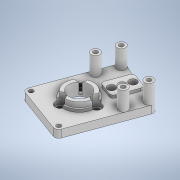
# Autodesk Inventor part: BASE_PLATE
Saved by Autodesk Inventor 2022 (Build 260153070, 153G)
## iProperties
Created: 2022-01-11
Part Number: BASE_PLATE
Material: Generic
Document SubType Name: Modeling
Designer: a laptop
Density: 1 g/cm^3
Appearance: Default
Author: a laptop
Autodesk Inventor part; units mm, degrees
ref_plane "YZ Plane" through (0, 0, 0) normal (1, 0, 0) x (0, 1, 0)
ref_plane "XZ Plane" through (0, 0, 0) normal (0, 1, 0) x (-1, 0, 0)
ref_plane "XY Plane" through (0, 0, 0) normal (0, 0, 1) x (1, 0, 0)
sketch "Sketch1" plane through (0, 0, 0) normal (0, 1, 0) x (-1, 0, 0)
  circle A0 centre (0, 0) radius 1.5
  circle A1 centre (-11.0608, 10.4718) radius 1.35 projected
  circle A2 centre (-15.2112, -0.7876) radius 1.35 projected
  circle A3 centre (11.0608, -10.4718) radius 1.35 projected
  circle A4 centre (15.2112, 0.7876) radius 1.35 projected
  line L0 (-13.5003, 11.3711) -> (-17.6507, 0.1117) projected
  line L1 (13.5003, -11.3711) -> (17.6507, -0.1117) projected
  arc A5 (-17.6507, 0.1117) -> (-15.7505, -3.331) centre (-15.2112, -0.7876) ccw projected
  arc A6 (-7.4411, -5.73) -> (-15.7505, -3.331) centre (-28.2044, -62.0577) ccw projected
  line L2 (-7.4411, -5.73) -> (1.9418, -9.1887) projected
  arc A7 (9.8203, -12.7568) -> (1.9418, -9.1887) centre (-18.8216, -65.5164) ccw projected
  arc A8 (9.8203, -12.7568) -> (13.5003, -11.3711) centre (11.0608, -10.4718) ccw projected
  circle A9 centre (-0.6847, 38.6203) radius 1.35
  circle A10 centre (25.5872, 28.936) radius 1.35
  line L3 (15.2112, 0.7876) -> (25.5872, 28.936) construction
  line L4 (25.5872, 28.936) -> (-0.6847, 38.6203) construction
  line L5 (-0.6847, 38.6203) -> (-11.0608, 10.4718) construction
  line L6 (-11.0608, 10.4718) -> (15.2112, 0.7876) construction
  circle A11 centre (-0.6847, 38.6203) radius 2.6
  circle A12 centre (25.5872, 28.936) radius 2.6
  line L7 (-13.5003, 11.3711) -> (-3.1243, 39.5196)
  line L8 (0.2145, 41.0599) -> (26.4865, 31.3756)
  line L9 (17.6507, -0.1117) -> (28.0267, 28.0368)
  circle A13 centre (6.9174, 18.7657) radius 6.25 projected
  dimension "d0" = 3
  dimension "d1" = 2.7
  dimension "d2" = 2.7
  dimension "d3" = 30
  dimension "d4" = 1.25
  constraints: 14 end point, 5 centre point, 5 coincident, 4 point on circle, 4 tangent, 2 perpendicular, 1 equal radius, 1 parallel
  measures "d0" diameter of A0
  measures "d1" diameter of A9
  measures "d2" diameter of A10
  measures "d3" distance between parallel lines of L6 L4
  measures "d4" radial gap between concentric circles of A9 A11
extrude "Extrusion1" add sketch "Sketch1" along normal blind 3
sketch "Sketch2" plane through (0, 0, 0) normal (0, -1, 0) x (1, 0, 0)
  circle A0 centre (-6.9174, 18.7657) radius 14.5
  circle A1 centre (-6.9174, 18.7657) radius 12 projected
  circle A2 centre (0, 0) radius 3.05
  circle A3 centre (0, 0) radius 1.5 projected
  line L0 (-1.7424, -2.5033) -> (-15.2011, 6.8649)
  line L1 (2.9503, -0.7734) -> (7.1087, 15.0886)
  circle A4 centre (-11.0608, -10.4718) radius 2.6
  circle A5 centre (-15.2112, 0.7876) radius 2.6
  circle A6 centre (-25.5872, 28.936) radius 2.6
  circle A7 centre (0.6847, 38.6203) radius 2.6
  circle A8 centre (11.0608, 10.4718) radius 2.6
  circle A9 centre (15.2112, -0.7876) radius 2.6
  circle A10 centre (-11.0608, -10.4718) radius 1.35 projected
  circle A11 centre (-15.2112, 0.7876) radius 1.35 projected
  circle A12 centre (-25.5872, 28.936) radius 1.35 projected
  circle A13 centre (0.6847, 38.6203) radius 1.35 projected
  circle A14 centre (11.0608, 10.4718) radius 1.35 projected
  circle A15 centre (15.2112, -0.7876) radius 1.35 projected
  circle A16 centre (1.7293, -4.6914) radius 1.15 projected
  circle A17 centre (-1.7293, 4.6914) radius 1.15 projected
  circle A18 centre (1.7293, -4.6914) radius 2.4
  arc A19 (7.1087, 15.0886) -> (4.1273, -4.7906) centre (97.7032, -8.6614) ccw
  arc A20 (-0.0305, -6.3233) -> (-15.2011, 6.8649) centre (-68.7061, -70.0029) ccw
  circle A21 centre (-6.9174, 18.7657) radius 12.35
  dimension "d7" = 2.5
  dimension "d8" = 6.1
  dimension "d10" = 1.25
  dimension "d13" = 1.25
  dimension "d14" = 0.35
  constraints: 12 centre point, 10 point on circle, 9 concentric, 8 tangent, 5 equal radius, 4 end point, 1 coincident
  measures "d7" radial gap between concentric circles of A0 A1
  measures "d8" diameter of A2
  measures "d10" radial gap between concentric circles of A4 A10
  measures "d13" radial gap between concentric circles of A16 A18
  measures "d14" radial gap between concentric circles of A1 A21
extrude "Extrusion2" add sketch "Sketch2" along normal blind 1.6 contours A0 A17 | A0 A17 L1 A2 L0 | L0 A2 A18 A20 | A19 A18 A2 L1 | A17 A0 | A0 A17 | A18 A2 | A4 | A5 | A6 | A7 | A8 | A9 | A16 picked at (3.6779, -4.407)
sketch "Sketch3" plane through (0, 3, 0) normal (0, 1, 0) x (1, 0, 0)
  circle A0 centre (-6.9174, -18.7657) radius 6.25 projected
  circle A1 centre (-6.9174, -18.7657) radius 9.5
  point P0 (0, 0)
  dimension "d15" = 19
  constraints: 1 centre point, 1 coincident
  measures "d15" diameter of A1
extrude "Extrusion3" add sketch "Sketch3" along normal blind 1.6
sketch "Sketch4" plane through (-6.9174, 4.6, 18.7657) normal (0, 1, 0) x (1, 0, 0)
  circle A0 centre (0, 0) radius 8.425
  circle A1 centre (0, 0) radius 6.25 projected
  point P0 (6.9174, 18.7657)
  dimension "d18" = 16.85
  constraints: 1 centre point, 1 concentric
  measures "d18" diameter of A0
extrude "Extrusion4" add sketch "Sketch4" along normal blind 3
sketch "Sketch5" plane through (-6.9174, 7.6, 18.7657) normal (0, 1, 0) x (1, 0, 0)
  circle A0 centre (-5.7568, 6.918) radius 1.6 projected
  circle A1 centre (-3.1128, -8.4445) radius 1.6 projected
  circle A2 centre (8.8696, 1.5265) radius 1.6 projected
  point P0 (6.9174, 18.7657)
extrude "Extrusion5" cut sketch "Sketch5" against normal up to surface (7.6 mm away)
sketch "Sketch6" plane through (-6.9174, 7.6, 18.7657) normal (0, 1, 0) x (1, 0, 0)
  circle A0 centre (-3.1128, -8.4445) radius 2.875
  circle A1 centre (-5.7568, 6.918) radius 2.875
  circle A2 centre (8.8696, 1.5265) radius 2.875
  arc A3 (-4.7015, -8.255) -> (-1.7812, -9.3315) centre (-3.1128, -8.4445) ccw projected
  arc A4 (-4.7983, 8.1992) -> (-7.1908, 6.2083) centre (-5.7568, 6.918) ccw projected
  arc A5 (9.4998, 0.0559) -> (8.9719, 3.1232) centre (8.8696, 1.5265) ccw projected
  point P0 (6.9174, 18.7657)
  dimension "d23" = 5.75
  constraints: 3 centre point, 3 concentric, 2 equal radius
  measures "d23" diameter of A1
extrude "Extrusion6" cut sketch "Sketch6" against normal blind 6.5
sketch "Sketch7" plane through (0, 3, 0) normal (0, 1, 0) x (1, 0, 0)
  circle A0 centre (0, 0) radius 1.875 projected
  circle A1 centre (1.7293, 4.6914) radius 1.15 projected
  circle A2 centre (-1.7293, -4.6914) radius 1.15 projected
  circle A3 centre (0, 0) radius 2.275
  line L0 (7.2185, 3.6805) -> (3.1891, -7.2505)
  line L1 (0.6208, -8.4353) -> (-5.9472, -6.0142)
  line L2 (-7.132, -3.4459) -> (-3.1026, 7.4851)
  line L3 (-0.5343, 8.6699) -> (6.0336, 6.2488)
  line L4 (7.4411, 5.73) -> (-1.9418, 9.1887) projected
  arc A4 (0.6208, -8.4353) -> (3.1891, -7.2505) centre (1.3125, -6.5588) ccw
  arc A5 (7.2185, 3.6805) -> (6.0336, 6.2488) centre (5.3419, 4.3722) ccw
  arc A6 (-0.5343, 8.6699) -> (-3.1026, 7.4851) centre (-1.2261, 6.7933) ccw
  arc A7 (-7.132, -3.4459) -> (-5.9472, -6.0142) centre (-5.2554, -4.1377) ccw
  dimension "d26" = 0.4
  dimension "d27" = 5.5
  dimension "d28" = 5.5
  dimension "d29" = 2.7
  dimension "d30" = 2
  constraints: 8 end point, 8 point on circle, 8 tangent, 5 centre point, 3 equal radius, 3 perpendicular, 1 collinear, 1 concentric, 1 point on line
  measures "d26" radial gap between concentric circles of A0 A3
  measures "d27" distance from line of L0 A3.centre
  measures "d28" distance from line of L2 point (0, 0)
  measures "d29" distance from line of A2.centre L1
  measures "d30" radius of A4
extrude "Extrusion7" add sketch "Sketch7" along normal blind 1.6 contours L0 A4 L1 A7 L2 A6 L3 A5
sketch "Sketch8" plane through (0, 4.6, 0) normal (0, 1, 0) x (1, 0, 0)
  circle A0 centre (1.7293, 4.6914) radius 2.3
  circle A1 centre (1.7293, 4.6914) radius 1.15 projected
  circle A2 centre (-1.7293, -4.6914) radius 2.3
  circle A3 centre (-1.7293, -4.6914) radius 1.15 projected
  point P0 (0, 0)
  dimension "d33" = 4.6
  dimension "d34" = 4.6
  constraints: 2 centre point, 2 concentric
  measures "d33" diameter of A0
  measures "d34" diameter of A2
extrude "Extrusion8" cut sketch "Sketch8" against normal blind 3.6 contours A0 | A1 | A2 | A3
sketch "Sketch9" plane through (-1.7293, 1, 4.6914) normal (0, 1, 0) x (1, 0, 0)
  circle A0 centre (0, 0) radius 1.15
  circle A1 centre (3.4587, 9.3828) radius 1.15
  circle A2 centre (3.4587, 9.3828) radius 2.3 projected
  circle A3 centre (0, 0) radius 2.3 projected
  point P0 (1.7293, 4.6914)
  dimension "d37" = 2.3
  constraints: 2 centre point, 2 concentric, 1 equal radius
  measures "d37" diameter of A1
extrude "Extrusion9" cut sketch "Sketch9" against normal blind 10 contours A0 | A1
sketch "Sketch10" plane through (0, 3, 0) normal (0, 1, 0) x (1, 0, 0)
  circle A0 centre (-11.0608, 10.4718) radius 2.6 projected
  circle A1 centre (-11.0608, 10.4718) radius 1.35 projected
  circle A2 centre (-15.2112, -0.7876) radius 2.6 projected
  circle A3 centre (-15.2112, -0.7876) radius 1.35 projected
  circle A4 centre (15.2112, 0.7876) radius 2.6 projected
  circle A5 centre (15.2112, 0.7876) radius 1.35 projected
  circle A6 centre (11.0608, -10.4718) radius 2.6 projected
  circle A7 centre (11.0608, -10.4718) radius 1.35 projected
  point P0 (0, 0)
extrude "Extrusion10" add sketch "Sketch10" along normal blind 11.32
sketch "Sketch11" plane through (-15.2112, 0, 0.7876) normal (0, -1, 0) x (1, 0, 0)
  arc A0 (15.1806, -7.1108) -> (0.0101, 6.0773) centre (-53.495, -70.7904) ccw projected
  arc A1 (22.3198, 14.3011) -> (0.0101, 6.0773) centre (8.2938, 17.9781) ccw projected
  arc A2 (22.3198, 14.3011) -> (19.3385, -5.5782) centre (112.9144, -9.449) ccw projected
  arc A3 (15.1806, -7.1108) -> (19.3385, -5.5782) centre (16.9405, -5.479) ccw projected
  line L0 (-11.2753, 30.588) -> (14.9966, 40.2723) projected
  line L1 (-2.4395, -0.8993) -> (-12.8156, 27.2492) projected
  circle A4 centre (0, 0) radius 2.6 projected
  line L2 (1.7109, -12.1587) -> (-2.4395, -0.8993) projected
  arc A5 (13.2694, -9.9762) -> (5.3909, -13.5444) centre (34.0328, -66.3039) ccw projected
  line L3 (22.6522, -6.5176) -> (13.2694, -9.9762) projected
  arc A6 (30.9617, -4.1185) -> (22.6522, -6.5176) centre (43.4156, -62.8452) ccw projected
  line L4 (28.7115, 10.5836) -> (32.8619, -0.6758) projected
  circle A7 centre (26.2719, 9.6843) radius 2.6 projected
  line L5 (18.3354, 38.7321) -> (28.7115, 10.5836) projected
  arc A8 (14.9966, 40.2723) -> (18.3354, 38.7321) centre (15.8959, 37.8328) ccw projected
  arc A9 (-12.8156, 27.2492) -> (-11.2753, 30.588) centre (-10.376, 28.1485) ccw projected
  arc A10 (5.3909, -13.5444) -> (1.7109, -12.1587) centre (4.1504, -11.2594) ccw projected
  arc A11 (32.8619, -0.6758) -> (30.9617, -4.1185) centre (30.4223, -1.5751) ccw projected
  point P0 (15.2112, -0.7876)
  constraints: 2 other
extrude "Extrusion11" add sketch "Sketch11" along normal up to surface (1.6 mm away)
body "Solid1"
